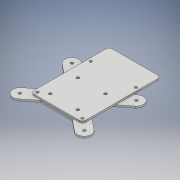
# Autodesk Inventor part: ChasisInferiorDron_P9
Saved by Autodesk Inventor 2017 (Build 210142000, 142)
## iProperties
Created: 2019-01-29
Part Number: ChasisInferiorDron_P9
Material: Generic
Document SubType Name: Modeling
Designer: Daniel Serena
Density: 1 g/cm^3
Appearance: Default
Author: Daniel Serena
Autodesk Inventor part; units mm, degrees
ref_plane "YZ Plane" through (0, 0, 0) normal (1, 0, 0) x (0, 1, 0)
ref_plane "XZ Plane" through (0, 0, 0) normal (0, 1, 0) x (-1, 0, 0)
ref_plane "XY Plane" through (0, 0, 0) normal (0, 0, 1) x (1, 0, 0)
sketch "Sketch1" plane through (0, 0, 0) normal (0, 0, 1) x (1, 0, 0)
  arc A0 (-38.9417, -24.6919) -> (-28.9986, -35.9017) centre (-34.2277, -30.5252) ccw
  arc A1 (40.4325, 20.1668) -> (31.0583, 31.8767) centre (35.7723, 26.0433) ccw
  arc A2 (-29.5767, 31.9271) -> (-38.9417, 20.21) centre (-34.2277, 26.0433) ccw
  arc A3 (31.0583, -36.3586) -> (40.1831, -24.4593) centre (35.7723, -30.5252) ccw
  line L0 (-16.5862, 21.6584) -> (18.4138, 21.6584)
  line L1 (-16.7484, -26.0092) -> (18.2516, -26.0092)
  line L2 (-20.4409, 5.259) -> (-20.4409, -9.741)
  line L3 (21.8055, 5.3953) -> (21.8055, -9.6047)
  circle A4 centre (-34.2277, 26.0433) radius 1.5
  circle A5 centre (35.7723, 26.0433) radius 1.5
  circle A6 centre (-34.2277, -30.5252) radius 1.5
  circle A7 centre (35.7723, -30.5252) radius 1.5
  circle A8 centre (-15.238, 13.5222) radius 1.5
  circle A9 centre (14.762, 13.5222) radius 1.5
  circle A10 centre (-15.238, -16.4778) radius 1.5
  circle A11 centre (14.762, -16.4778) radius 1.5
  line L4 (-34.2277, 26.0433) -> (-34.2277, 24.5433)
  line L5 (-34.2277, -29.0252) -> (-34.2277, -30.5252)
  line L6 (-38.9417, 20.21) -> (-20.4409, 5.259)
  line L7 (18.2516, -26.0092) -> (31.0583, -36.3586)
  line L8 (-15.238, 13.5222) -> (-15.238, 12.0222)
  line L9 (-15.238, -14.9778) -> (-15.238, -16.4778)
  line L10 (-38.9417, -24.6919) -> (-20.4409, -9.741)
  line L11 (35.7723, 26.0433) -> (35.7723, 24.5433)
  line L12 (34.2723, 26.0433) -> (35.7723, 26.0433)
  line L13 (40.7786, -24.9407) -> (21.8055, -9.6047)
  line L14 (-16.5862, 21.6584) -> (-29.5767, 31.9271)
  line L15 (-15.238, 15.0222) -> (-15.238, 13.5222)
  line L16 (18.4138, 21.6584) -> (31.0583, 31.8767)
  line L17 (-15.238, 13.5222) -> (-13.738, 13.5222)
  line L18 (13.262, 13.5222) -> (14.762, 13.5222)
  line L19 (14.762, 13.5222) -> (14.762, 12.0222)
  line L20 (14.762, -14.9778) -> (14.762, -16.4778)
  line L21 (14.762, -16.4778) -> (13.262, -16.4778)
  line L22 (-13.738, -16.4778) -> (-15.238, -16.4778)
  line L23 (-28.9986, -35.9017) -> (-16.7484, -26.0092)
  line L24 (21.8055, 5.3953) -> (40.4325, 20.1668)
  line L25 (35.7723, -30.5252) -> (34.2723, -30.5252)
  line L26 (-32.7277, -30.5252) -> (-34.2277, -30.5252)
  line L27 (35.7723, -29.0252) -> (35.7723, -30.5252)
  dimension "d27" = 3
  dimension "d6" = 15
  dimension "d7" = 15
  dimension "d9" = 15
  dimension "d10" = 15
  dimension "d16" = 90
  dimension "d17" = 90
  dimension "d20" = 70
  dimension "d23" = 35
  dimension "d24" = 35
  dimension "d25" = 15
  dimension "d26" = 15
  dimension "d28" = 3
  dimension "d29" = 3
  dimension "d30" = 3
  dimension "d33" = 30
  dimension "d35" = 30
  dimension "d37" = 30
  dimension "d39" = 3
  dimension "d40" = 3
  dimension "d41" = 3
  dimension "d42" = 3
  dimension "d45" = 70
  dimension "d46" = 56.5685
  dimension "d47" = 56.5685
  constraints: 56 end point, 24 point on circle, 14 perpendicular, 12 tangent, 11 centre point, 8 coincident, 4 vertical, 3 horizontal, 1 point on line, 1 vertical alignment, 2 other
  measures "d6" diameter of A0
  measures "d7" diameter of A1
  measures "d9" diameter of A2
  measures "d10" diameter of A3
  measures "d16" distance of L25.start L4.start
  measures "d17" distance of L11.start L5.end
  measures "d20" distance of L25.start L5.end
  measures "d23" distance of L0.start L0.end
  measures "d24" distance of L1.end L1.start
  measures "d25" distance of L2.start L2.end
  measures "d26" distance of L3.end L3.start
  measures "d28" diameter of A5
  measures "d29" diameter of A6
  measures "d30" diameter of A7
  measures "d33" distance of L8.start L18.end
  measures "d35" distance of L18.end L20.end
  measures "d37" distance of L20.end L9.end
  measures "d39" diameter of A8
  measures "d40" diameter of A9
  measures "d41" diameter of A10
  measures "d42" diameter of A11
  measures "d45" distance of L11.start L4.start
  measures "d46" distance of L4.start L5.end
  measures "d47" distance of L25.start A5.centre
extrude "Extrusion1" add sketch "Sketch1" along normal blind 2 contours L10 L2 L6 A2 L14 L0 L16 A1 L24 L3 L13 A3 L7 L1 L23 A0
sketch "Sketch2" plane through (0, 0, 2) normal (0, 0, 1) x (1, 0, 0)
  line L0 (-23.7277, 59.388) -> (25.2723, 59.388)
  line L1 (25.2723, -25.5399) -> (-23.7277, -25.5399)
  arc A0 (-23.7277, 59.388) -> (-27.2277, 55.888) centre (-23.7277, 55.888) ccw
  arc A1 (28.7723, 55.888) -> (25.2723, 59.388) centre (25.2723, 55.888) ccw
  arc A2 (-27.2277, -22.0399) -> (-23.7277, -25.5399) centre (-23.7277, -22.0399) ccw
  arc A3 (25.2723, -25.5399) -> (28.7723, -22.0399) centre (25.2723, -22.0399) ccw
  circle A4 centre (-23.7277, -22.0399) radius 1.375
  circle A5 centre (25.2723, -22.0399) radius 1.375
  circle A6 centre (-34.2277, -30.5252) radius 1.5 projected
  circle A7 centre (-34.2277, 26.0433) radius 1.5 projected
  circle A8 centre (35.7723, 26.0433) radius 1.5 projected
  circle A9 centre (-15.238, -16.4778) radius 1.5 projected
  circle A10 centre (14.762, -16.4778) radius 1.5 projected
  circle A11 centre (14.762, 13.5222) radius 1.5 projected
  circle A12 centre (35.7723, -30.5252) radius 1.5 projected
  circle A13 centre (-34.2277, -30.5252) radius 1.5 projected
  line L2 (40.7786, -24.9407) -> (21.8055, -9.6047) projected
  line L3 (21.8055, -9.6047) -> (21.8055, 5.3953) projected
  line L4 (21.8055, 5.3953) -> (40.4325, 20.1668) projected
  arc A14 (40.4325, 20.1668) -> (31.0583, 31.8767) centre (35.7723, 26.0433) ccw projected
  line L5 (31.0583, 31.8767) -> (18.4138, 21.6584) projected
  line L6 (18.4138, 21.6584) -> (-16.5862, 21.6584) projected
  line L7 (-16.5862, 21.6584) -> (-29.5767, 31.9271) projected
  arc A15 (-29.5767, 31.9271) -> (-38.9417, 20.21) centre (-34.2277, 26.0433) ccw projected
  line L8 (-38.9417, 20.21) -> (-20.4409, 5.259) projected
  line L9 (-20.4409, 5.259) -> (-20.4409, -9.741) projected
  line L10 (-20.4409, -9.741) -> (-38.9417, -24.6919) projected
  arc A16 (-38.9417, -24.6919) -> (-28.9986, -35.9017) centre (-34.2277, -30.5252) ccw projected
  line L11 (-28.9986, -35.9017) -> (-16.7484, -26.0092) projected
  line L12 (-16.7484, -26.0092) -> (18.2516, -26.0092) projected
  line L13 (18.2516, -26.0092) -> (31.0583, -36.3586) projected
  arc A17 (31.0583, -36.3586) -> (40.7786, -24.9407) centre (35.7723, -30.5252) ccw projected
  circle A18 centre (-15.238, 13.5222) radius 1.5 projected
  circle A19 centre (35.7723, 26.0433) radius 1.5 projected
  circle A20 centre (-34.2277, 26.0433) radius 1.5 projected
  circle A21 centre (-23.7277, 35.9601) radius 1.375
  circle A22 centre (25.2723, 35.9601) radius 1.375
  line L14 (28.7723, 55.888) -> (28.7723, -22.0399)
  line L15 (28.7723, -24.8684) -> (28.7723, -25.5399)
  line L16 (-27.2277, -25.5399) -> (-27.2277, -24.8684)
  line L17 (-27.2277, -22.0399) -> (-27.2277, 55.888)
  line L18 (34.6056, 25.1005) -> (35.7723, 26.0433)
  line L19 (-34.2277, 26.0433) -> (-33.061, 25.1005)
  line L20 (-34.2277, -30.5252) -> (-33.061, -29.5824)
  line L21 (-27.2277, -24.8684) -> (-22.6582, -21.1757)
  line L22 (27.9945, -24.2398) -> (28.7723, -24.8684)
  line L23 (34.6056, -29.5824) -> (35.7723, -30.5252)
  point P0 (0, 0)
  dimension "d54" = 2.75
  dimension "d48" = 56
  dimension "d49" = 85
  dimension "d50" = 7
  dimension "d51" = 7
  dimension "d52" = 7
  dimension "d53" = 7
  dimension "d55" = 2.75
  dimension "d56" = 2.75
  dimension "d57" = 2.75
  dimension "d58" = 58
  dimension "d59" = 58
  constraints: 24 end point, 12 tangent, 9 point on circle, 7 centre point, 5 parallel, 2 coincident, 2 perpendicular, 2 vertical alignment, 1 horizontal, 1 point on line, 11 other
  measures "d48" distance of L15.end L16.start
  measures "d49" distance of L0.end L15.end
  measures "d50" diameter of A0
  measures "d51" diameter of A1
  measures "d52" diameter of A2
  measures "d53" diameter of A3
  measures "d55" diameter of A5
  measures "d56" diameter of A21
  measures "d57" diameter of A22
  measures "d58" distance of A2.centre A21.centre
  measures "d59" distance of A3.centre A22.centre
extrude "Extrusion2" add sketch "Sketch2" along normal blind 2 contours L0 A1 L14 L5 L6 L7 L17 A0 | L7 L6 L5 L14 L4 L3 L2 A3 L1 A2 L17 L10 L9 L8 | L8 L9 L10 L17 | L14 L2 L3 L4
hole "Hole1" at (-23.7277, -22.0399, 4) direction (0, 0, -1) diameter 3 end through all
hole "Hole2" at (25.2723, -22.0399, 2) direction (0, 0, -1) diameter 3 end through all
equation "\"d24\" = d23"
body "Solid1"
